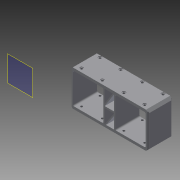
# Autodesk Inventor part: 2 cam holder 0.1 tolerance
Saved by Autodesk Inventor 2015 (Build 190159000, 159)
## iProperties
Created: 2015-03-12
Part Number: 2 cam holder 0.1 tolerance
Material: Nylon 6/6
Document SubType Name: Modeling
Designer: Vladimir
Density: 1.13 g/cm^3
Appearance: Nylon 6
Author: Vladimir
Autodesk Inventor part; units mm, degrees
ref_plane "YZ Plane" through (0, 0, 0) normal (1, 0, 0) x (0, 1, 0)
ref_plane "XZ Plane" through (0, 0, 0) normal (0, 1, 0) x (-1, 0, 0)
ref_plane "XY Plane" through (0, 0, 0) normal (0, 0, 1) x (1, 0, 0)
ref_plane "Work Plane11" through (-14.365, -0.3025, 0) normal (0, 0, -1) x (-1, 0, 0)
sketch "0.1 tolerance" plane through (-14.365, -0.3025, 0) normal (0, 0, -1) x (-1, 0, 0)
  line L0 (-111.2019, 0.0288) -> (-111.2019, 27.0288)
  line L1 (-83.7019, 0.2788) -> (-107.8019, 0.2788)
  line L2 (-109.0019, 1.4788) -> (-109.0019, 25.5788)
  line L3 (-107.8019, 26.7788) -> (-83.7019, 26.7788)
  line L4 (-82.5019, 25.5788) -> (-82.5019, 1.4788)
  line L5 (-71.1019, 0.2288) -> (-47.0019, 0.2288)
  line L6 (-45.8019, 1.4288) -> (-45.8019, 25.5788)
  line L7 (-47.0019, 26.7788) -> (-71.1019, 26.7788)
  line L8 (-72.3019, 25.5788) -> (-72.3019, 1.4288)
  line L9 (-43.6019, 0.0288) -> (-43.6019, 27.0288)
  line L10 (-109.2019, -1.9712) -> (-45.6019, -1.9712)
  line L11 (-109.2019, 29.0288) -> (-45.6019, 29.0288)
  line L12 (-81.5019, 12.3053) -> (-73.3019, 0.2288)
  line L13 (-74.5107, 0.2288) -> (-81.5019, 10.5251)
  line L14 (-74.5107, 0.2288) -> (-81.5019, 0.2288)
  line L15 (-73.3019, 0.2288) -> (-73.3019, 12.3053)
  line L16 (-81.5019, 10.5251) -> (-81.5019, 0.2288)
  line L17 (-81.5019, 12.3053) -> (-73.3019, 12.3053)
  arc A0 (-71.1019, 26.7788) -> (-72.3019, 25.5788) centre (-71.1019, 25.5788) ccw
  arc A1 (-72.3019, 1.4288) -> (-71.1019, 0.2288) centre (-71.1019, 1.4288) ccw
  arc A2 (-47.0019, 0.2288) -> (-45.8019, 1.4288) centre (-47.0019, 1.4288) ccw
  arc A3 (-45.8019, 25.5788) -> (-47.0019, 26.7788) centre (-47.0019, 25.5788) ccw
  arc A4 (-107.8019, 26.7788) -> (-109.0019, 25.5788) centre (-107.8019, 25.5788) ccw
  arc A5 (-82.5019, 25.5788) -> (-83.7019, 26.7788) centre (-83.7019, 25.5788) ccw
  arc A6 (-83.7019, 0.2788) -> (-82.5019, 1.4788) centre (-83.7019, 1.4788) ccw
  arc A7 (-109.0019, 1.4788) -> (-107.8019, 0.2788) centre (-107.8019, 1.4788) ccw
  line L18 (-45.6019, -1.9712) -> (-43.6019, 0.0288)
  line L19 (-45.6019, 29.0288) -> (-43.6019, 27.0288)
  line L20 (-111.2019, 0.0288) -> (-109.2019, -1.9712)
  line L21 (-109.2019, 29.0288) -> (-111.2019, 27.0288)
  line L22 (-80.3189, 26.7788) -> (-73.3019, 26.7788)
  line L23 (-81.5019, 26.7788) -> (-81.5019, 13.8053)
  line L24 (-80.3189, 26.7788) -> (-73.3019, 15.6769)
  line L25 (-73.3019, 15.6769) -> (-73.3019, 26.7788)
  line L26 (-73.3019, 13.8053) -> (-81.5019, 26.7788)
  line L27 (-73.3019, 13.8053) -> (-81.5019, 13.8053)
  point P0 (-70.0019, 0.2767)
  point P1 (-111.2019, 29.0288)
  point P2 (-111.2019, -1.9712)
  point P3 (-82.5019, 0.2788)
  point P4 (-109.0019, 26.7788)
  point P5 (-109.0019, 0.2788)
  point P6 (-82.5019, 26.7788)
  point P7 (-45.8019, 26.7788)
  point P8 (-72.3019, 26.7788)
  point P9 (-43.6019, 29.0288)
  point P10 (-43.6019, -1.9712)
  dimension "d368" = 31
  dimension "d366" = 26.5
  dimension "d367" = 26.5
  dimension "d364" = 26.5
  dimension "d361" = 2.2
  dimension "d365" = 2.2
  dimension "d362" = 67.6
  dimension "d353" = 1.2
  dimension "d352" = 1.2
  dimension "d351" = 1.2
  dimension "d350" = 1.2
  dimension "d349" = 1.2
  dimension "d348" = 1.2
  dimension "d347" = 1.2
  dimension "d346" = 1.2
  dimension "d345" = 2
  dimension "d344" = 2
  dimension "d343" = 2
  dimension "d342" = 2
  dimension "d341" = 2
  dimension "d340" = 2
  dimension "d339" = 2
  dimension "d338" = 2
  dimension "d363" = 26.55
  dimension "d355" = 1
  dimension "d357" = 1
  dimension "d356" = 2.2
  dimension "d360" = 2.25
  dimension "d372" = 2.25
  dimension "d354" = 1
  dimension "d373" = 10.2
  dimension "d358" = 2.2
  dimension "d337" = 2.25
  dimension "d336" = 2.25
  dimension "d331" = 1.5
  dimension "d333" = 1
  dimension "d359" = 1
  dimension "d335" = 1
  dimension "d334" = 1
  dimension "d332" = 1
  dimension "d410" = 2.25
  constraints: 56 end point, 20 point on line, 16 point on circle, 16 tangent, 8 centre point, 6 parallel, 6 perpendicular, 5 horizontal, 1 vertical
  measures "d368" distance of point (-111.202, -1.971) point (-111.202, 29.029)
  measures "d366" distance of point (-109.002, 26.779) point (-82.502, 26.779)
  measures "d367" distance of point (-109.002, 0.279) point (-109.002, 26.779)
  measures "d364" distance of point (-72.302, 26.779) point (-45.802, 26.779)
  measures "d361" distance between parallel lines of L9 L6
  measures "d365" distance between parallel lines of L0 L2
  measures "d362" distance of point (-111.202, 29.029) point (-43.602, 29.029)
  measures "d353" radius of A0
  measures "d352" radius of A1
  measures "d351" radius of A2
  measures "d350" radius of A3
  measures "d349" radius of A4
  measures "d348" radius of A5
  measures "d347" radius of A6
  measures "d346" radius of A7
  measures "d345" distance of L10.end point (-43.602, -1.971)
  measures "d344" distance of L9.start point (-43.602, -1.971)
  measures "d343" distance of L11.end point (-43.602, 29.029)
  measures "d342" distance of L9.end point (-43.602, 29.029)
  measures "d341" distance of L0.start point (-111.202, -1.971)
  measures "d340" distance of L10.start point (-111.202, -1.971)
  measures "d339" distance of L11.start point (-111.202, 29.029)
  measures "d338" distance of L0.end point (-111.202, 29.029)
  measures "d363" distance between parallel lines of L5 L7
  measures "d355" distance between parallel lines of L8 L15
  measures "d357" distance between parallel lines of L12 L13
  measures "d356" distance between parallel lines of L10 L14
  measures "d360" distance between parallel lines of L3 L11
  measures "d372" distance between parallel lines of L10 L1
  measures "d354" distance between parallel lines of L4 L16
  measures "d373" distance between parallel lines of L8 L4
  measures "d358" distance from line of L10 L12.end
  measures "d337" distance from line of L11 L23.start
  measures "d336" distance between parallel lines of L11 L22
  measures "d331" distance between parallel lines of L17 L27
  measures "d333" distance between parallel lines of L24 L26
  measures "d359" distance from line of L4 L12.start
  measures "d335" distance between parallel lines of L4 L23
  measures "d334" distance between parallel lines of L8 L25
  measures "d332" distance from line of L8 L26.start
  measures "d410" distance between parallel lines of L7 L11
extrude "0.1 mm tolerance" add sketch "0.1 tolerance" along normal blind 21
sketch "Sketch11" plane through (65.037, 28.7262, -10.5) normal (0, 1, 0) x (1, 0, 0)
  line L0 (-35.8, 10.5) -> (31.8, 10.5)
  line L1 (31.8, 10.5) -> (31.8, -10.5)
  line L2 (31.8, -10.5) -> (-35.8, -10.5)
  line L3 (-35.8, -10.5) -> (-35.8, 10.5)
  line L4 (-33.8499, -10.5) -> (29.7501, -10.5)
  line L5 (-35.8, 10.5) -> (-33.55, 10.5)
  line L6 (-33.55, 10.5) -> (-33.55, -10.5)
  line L7 (-33.55, -10.5) -> (-35.8, -10.5)
  line L8 (-35.8, -10.5) -> (-35.8, 10.5)
  line L9 (-33.55, 10.5) -> (-7.15, 10.5)
  line L10 (-7.15, 10.5) -> (-7.15, -10.5)
  line L11 (-7.15, -10.5) -> (-33.55, -10.5)
  line L12 (-33.55, -10.5) -> (-33.55, 10.5)
  line L13 (31.8, -10.5) -> (29.55, -10.5)
  line L14 (29.55, -10.5) -> (29.55, 10.5)
  line L15 (29.55, 10.5) -> (31.8, 10.5)
  line L16 (31.8, 10.5) -> (31.8, -10.5)
  line L17 (-33.9719, 10.5) -> (29.6281, 10.5)
  line L18 (29.55, -10.5) -> (3.15, -10.5)
  line L19 (3.15, -10.5) -> (3.15, 10.5)
  line L20 (3.15, 10.5) -> (29.55, 10.5)
  line L21 (29.55, 10.5) -> (29.55, -10.5)
  circle A0 centre (25.35, 8.8) radius 0.95
  circle A1 centre (7.35, 8.8) radius 0.95
  circle A2 centre (25.3501, -7.2) radius 0.95
  circle A3 centre (7.3501, -7.2) radius 0.95
  circle A4 centre (-11.35, 8.8) radius 0.95
  circle A5 centre (-29.35, 8.8) radius 0.95
  circle A6 centre (-29.35, -7.2) radius 0.95
  circle A7 centre (-11.35, -7.2) radius 0.95
  point P0 (5.2281, 10.5)
  dimension "d400" = 2.25
  dimension "d399" = 26.4
  dimension "d398" = 2.25
  dimension "d397" = 26.4
  dimension "d394" = 1.9
  dimension "d391" = 1.9
  dimension "d393" = 18
  dimension "d396" = 4.2
  dimension "d392" = 4.2
  dimension "d395" = 1.7
  dimension "d389" = 1.9
  dimension "d387" = 1.9
  dimension "d390" = 16
  dimension "d388" = 16
  dimension "d384" = 1.9
  dimension "d381" = 1.9
  dimension "d378" = 1.9
  dimension "d375" = 1.9
  dimension "d377" = 16
  dimension "d386" = 1.7
  dimension "d383" = 1.7
  dimension "d382" = 18
  dimension "d385" = 4.2
  dimension "d407" = 4.2
  dimension "d376" = 4.2
  dimension "d380" = 4.2
  dimension "d379" = 16
  dimension "d408" = 18
  dimension "d409" = 67.6
  constraints: 44 end point, 10 parallel, 8 centre point, 5 horizontal, 5 perpendicular, 4 point on line
  measures "d400" distance of L6.end L7.end
  measures "d399" distance of L10.end L11.end
  measures "d398" distance of L14.end L15.end
  measures "d397" distance of L19.end L20.end
  measures "d394" diameter of A0
  measures "d391" diameter of A1
  measures "d393" distance of A1.centre A0.centre
  measures "d396" distance from line of A0.centre L21
  measures "d392" distance from line of L19 A1.centre
  measures "d395" distance from line of L20 A0.centre
  measures "d389" diameter of A2
  measures "d387" diameter of A3
  measures "d390" distance of A0.centre A2.centre
  measures "d388" distance of A1.centre A3.centre
  measures "d384" diameter of A4
  measures "d381" diameter of A5
  measures "d378" diameter of A6
  measures "d375" diameter of A7
  measures "d377" distance of A7.centre A4.centre
  measures "d386" distance from line of L9 A4.centre
  measures "d383" distance from line of L9 A5.centre
  measures "d382" distance of A4.centre A5.centre
  measures "d385" distance from line of L10 A4.centre
  measures "d407" distance from line of L6 A5.centre
  measures "d376" distance from line of L10 A7.centre
  measures "d380" distance from line of L6 A6.centre
  measures "d379" distance of A5.centre A6.centre
  measures "d408" distance of A6.centre A7.centre
  measures "d409" distance between parallel lines of L8 L1
hole "Hole7" at (29.237, 28.7262, -21) at (90.387, 28.7262, -19.3) at (90.3871, 28.7262, -3.3) at (72.3871, 28.7262, -3.3) at (72.387, 28.7262, -19.3) at (53.687, 28.7262, -3.3) at (53.687, 28.7262, -19.3) at (35.687, 28.7262, -3.3) at (35.687, 28.7262, -19.3) at (29.237, 28.7262, 0) at (96.837, 28.7262, 0) at (96.837, 28.7262, -21) direction (0, -1, 0) diameter 1.9 end through all counterbore diameter 3 counterbore depth 0.5
body "Solid1"
